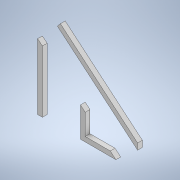
# Autodesk Inventor part: newFrameV02
Saved by Autodesk Inventor 2020.2 (Build 242310000, 310)
## iProperties
Created: 2020-02-22
Part Number: newFrameV02
Material: Generic
Document SubType Name: Modeling
Designer: robst
Density: 1 g/cm^3
Appearance: Default
Author: robst
Autodesk Inventor part; units mm, degrees
ref_plane "YZ Plane" through (0, 0, 0) normal (1, 0, 0) x (0, 1, 0)
ref_plane "XZ Plane" through (0, 0, 0) normal (0, 1, 0) x (-1, 0, 0)
ref_plane "XY Plane" through (0, 0, 0) normal (0, 0, 1) x (1, 0, 0)
sketch "Sketch1" plane through (0, 0, 0) normal (0, 0, 1) x (1, 0, 0)
  line L0 (0, 0) -> (-228.6, 0) construction
  line L1 (0, 0) -> (-39.5154, 0)
  line L2 (-457.2, 350.479) -> (-457.2, 0)
  line L3 (-431.8, 329.1659) -> (-431.8, 0)
  line L4 (-228.6, 158.6608) -> (-228.6, 0)
  line L5 (-203.2, 137.3477) -> (-203.2, 0)
  line L6 (-457.2, 0) -> (-431.8, 0)
  line L7 (-228.6, 0) -> (-203.2, 0)
  line L8 (-203.2, 0) -> (-39.5154, 0)
  line L9 (-203.2, 25.4) -> (-69.7859, 25.4)
  line L10 (-351.8656, 461.0371) -> (76.2, 101.8473)
  line L11 (76.2, 135.0047) -> (-335.5388, 480.4946)
  line L12 (-335.5388, 480.4946) -> (-351.8656, 461.0371)
  line L13 (0, 0) -> (0, 391.6762) construction
  line L14 (76.2, 135.0047) -> (76.2, 101.8473)
  line L15 (-431.8, 329.1659) -> (-457.2, 350.479)
  line L16 (-39.5154, 0) -> (-69.7859, 25.4)
  line L17 (-203.2, 137.3477) -> (-228.6, 158.6608)
  dimension "d19" = 25.4
  dimension "d21" = 25.4
  dimension "d27" = 25.4
  dimension "d29" = 76.2
  dimension "d30" = 558.8
  dimension "d31" = 25.4
  constraints: 36 end point, 6 perpendicular, 6 point on line, 2 horizontal, 2 vertical, 1 collinear, 1 parallel
  measures "d19" distance between parallel lines of L3 L2
  measures "d21" distance between parallel lines of L5 L4
  measures "d27" distance between parallel lines of L9 L8
  measures "d29" distance between parallel lines of L14 L13
  measures "d30" distance of L10.start L10.end
  measures "d31" distance between parallel lines of L11 L10
extrude "Extrusion1" add sketch "Sketch1" along normal mid plane 25.4
body "Solid1"
